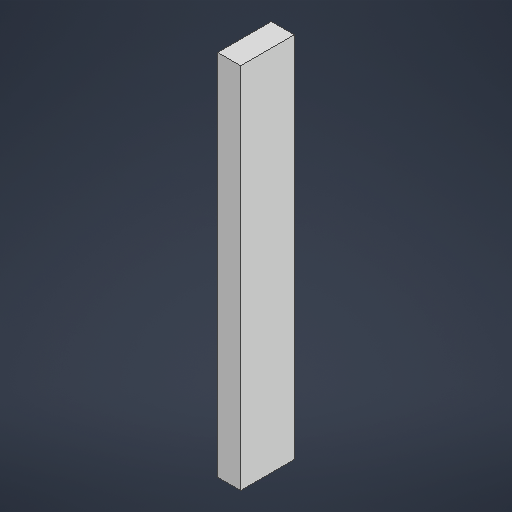
# Autodesk Inventor part: 2x4x30
Saved by Autodesk Inventor 2027.1 (Build 311270010, 270A)
## iProperties
Created: 2026-08-30
Part Number: 2x4x30
Material: Generic
Document SubType Name: Modeling
Designer: jorda
Density: 1 g/cm^3
Appearance: Default
Author: jorda
Autodesk Inventor part; units mm, degrees
ref_plane "YZ Plane" through (0, 0, 0) normal (1, 0, 0) x (0, 1, 0)
ref_plane "XZ Plane" through (0, 0, 0) normal (0, 1, 0) x (-1, 0, 0)
ref_plane "XY Plane" through (0, 0, 0) normal (0, 0, 1) x (1, 0, 0)
sketch "Sketch1" plane through (0, 0, 0) normal (0, 1, 0) x (-1, 0, 0)
  line L0 (19.05, 44.45) -> (-19.05, 44.45)
  line L1 (-19.05, 44.45) -> (-19.05, -44.45)
  line L2 (-19.05, -44.45) -> (19.05, -44.45)
  line L3 (19.05, -44.45) -> (19.05, 44.45)
  line L4 (19.05, 44.45) -> (-19.05, -44.45) construction
  line L5 (-19.05, 44.45) -> (19.05, -44.45) construction
  point P0 (0, 0)
  dimension "d1" = 38.1
  dimension "d2" = 88.9
  constraints: 12 end point, 2 midpoint, 2 parallel, 1 horizontal, 1 perpendicular
  measures "d1" distance of L2.end L1.end
  measures "d2" distance of L1.end L0.end
extrude "Extrusion1" add sketch "Sketch1" along normal blind 609.6
body "Solid1"
